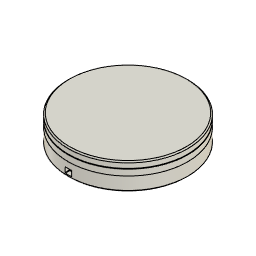
Turntable v8 (Autodesk Fusion 360 design; units mm, degrees)
Autodesk Fusion 360 part; units mm, degrees
sketch "Skizze1" plane through (0, 0, 0) normal (0, 0, 1) x (1, 0, 0)
  circle A0 centre (0, 0) radius 100
  circle A1 centre (0, 0) radius 86
  circle A2 centre (0, 0) radius 9
  dimension "d1" = 200
  dimension "d145" = 172
  dimension "d147" = 18
  constraint coincident A0.centre A1.centre
  constraint concentric A0 A2
  measures "d1" diameter of A0
  measures "d145" diameter of A1
  measures "d147" diameter of A2
extrude "Extrusion1" add sketch "Skizze1" along normal blind 10 from surface at 0.5 contours A0 | A1 | A2 makes body 1
chamfer "Fase1" distance 2 angle 45 1 edges at (-93.2327, -36.1615, 10.5) on bodies 1
sketch "Skizze2" plane through (0, 0, 0) normal (0, 1, 0) x (1, 0, 0)
  circle A0 centre (-93, 0) radius 3.5
  line L0 (0, 0) -> (-93, 0) construction
  dimension "d6" = 7
  dimension "d8" = 93
  constraint coincident L0.start origin
  constraint coincident A0.centre L0.end
  constraint horizontal L0
  measures "d6" diameter of A0
  measures "d8" distance of L0.start A0.centre
revolve "Drehen1" cut sketch "Skizze2" angle 360 about axis through (0, 0, 1.75) along (0, 0, 1) bodies 1
sketch "Skizze3" plane through (0, 0, 0) normal (0, 0, 1) x (1, 0, 0)
  circle A0 centre (0, 0) radius 100
  circle A1 centre (0, 0) radius 85
  line L0 (-3.8, 94) -> (-3.8, 91)
  arc A2 (-3.8, 91) -> (3.8, 91) centre (0, 91) ccw
  line L1 (3.8, 91) -> (3.8, 94)
  arc A3 (3.8, 94) -> (-3.8, 94) centre (0, 94) ccw
  line L2 (0, 94) -> (0, 91) construction
  line L3 (0, 0) -> (0, 94) construction
  line L4 (0, 0) -> (81.4064, 47) construction
  line L5 (79.5064, 50.2909) -> (76.9083, 48.7909)
  arc A4 (76.9083, 48.7909) -> (80.7083, 42.2091) centre (78.8083, 45.5) ccw
  line L6 (80.7083, 42.2091) -> (83.3064, 43.7091)
  arc A5 (83.3064, 43.7091) -> (79.5064, 50.2909) centre (81.4064, 47) ccw
  line L7 (81.4064, 47) -> (78.8083, 45.5) construction
  line L8 (0, 0) -> (81.4064, -47) construction
  line L9 (0, 0) -> (0, -94) construction
  line L10 (0, 0) -> (-81.4064, -47) construction
  line L11 (0, 0) -> (-81.4064, 47) construction
  line L12 (83.3064, -43.7091) -> (80.7083, -42.2091)
  arc A6 (80.7083, -42.2091) -> (76.9083, -48.7909) centre (78.8083, -45.5) ccw
  line L13 (76.9083, -48.7909) -> (79.5064, -50.2909)
  arc A7 (79.5064, -50.2909) -> (83.3064, -43.7091) centre (81.4064, -47) ccw
  line L14 (81.4064, -47) -> (78.8083, -45.5) construction
  line L15 (3.8, -94) -> (3.8, -91)
  arc A8 (3.8, -91) -> (-3.8, -91) centre (0, -91) ccw
  line L16 (-3.8, -91) -> (-3.8, -94)
  arc A9 (-3.8, -94) -> (3.8, -94) centre (0, -94) ccw
  line L17 (0, -94) -> (0, -91) construction
  line L18 (-79.5064, -50.2909) -> (-76.9083, -48.7909)
  arc A10 (-76.9083, -48.7909) -> (-80.7083, -42.2091) centre (-78.8083, -45.5) ccw
  line L19 (-80.7083, -42.2091) -> (-83.3064, -43.7091)
  arc A11 (-83.3064, -43.7091) -> (-79.5064, -50.2909) centre (-81.4064, -47) ccw
  line L20 (-81.4064, -47) -> (-78.8083, -45.5) construction
  line L21 (-83.3064, 43.7091) -> (-80.7083, 42.2091)
  arc A12 (-80.7083, 42.2091) -> (-76.9083, 48.7909) centre (-78.8083, 45.5) ccw
  line L22 (-76.9083, 48.7909) -> (-79.5064, 50.2909)
  arc A13 (-79.5064, 50.2909) -> (-83.3064, 43.7091) centre (-81.4064, 47) ccw
  line L23 (-81.4064, 47) -> (-78.8083, 45.5) construction
  dimension "d10" = 200
  dimension "d11" = 170
  dimension "d138" = 3.8
  dimension "d139" = 3
  dimension "d140" = 94
  dimension "d141" = 60
  dimension "d142" = 60
  constraint coincident A0.centre A1.centre
  constraint tangent L0 A2
  constraint tangent A2 L1
  constraint parallel L0 L1
  constraint tangent L1 A3
  constraint tangent L0 A3
  constraint coincident A3.centre L2.start
  constraint coincident A2.centre L3
  constraint vertical L3
  constraint tangent L5 A4
  constraint tangent A4 L6
  constraint parallel L5 L6
  constraint tangent L6 A5
  constraint tangent L5 A5
  constraint coincident L4 A4.centre
  constraint parallel L4 L7
  constraint coincident L4.end A5.centre
  constraint equal L1 L5
  constraint equal A3 A5
  constraint equal L3 L4
  constraint parallel L3 L9
  constraint parallel L8 L11
  constraint parallel L4 L10
  constraint equal L4 L8
  constraint equal L8 L9
  constraint equal L9 L10
  constraint equal L10 L11
  constraint tangent L12 A6
  constraint tangent A6 L13
  constraint parallel L12 L13
  constraint tangent L13 A7
  constraint tangent L12 A7
  constraint coincident L8 A6.centre
  constraint parallel L8 L14
  constraint coincident L8.end A7.centre
  constraint tangent L15 A8
  constraint tangent A8 L16
  constraint parallel L15 L16
  constraint tangent L16 A9
  constraint tangent L15 A9
  constraint coincident L9 A8.centre
  constraint parallel L9 L17
  constraint coincident L9.end A9.centre
  constraint tangent L18 A10
  constraint tangent A10 L19
  constraint parallel L18 L19
  constraint tangent L19 A11
  constraint tangent L18 A11
  constraint coincident L10 A10.centre
  constraint parallel L10 L20
  constraint coincident L10.end A11.centre
  constraint tangent L21 A12
  constraint tangent A12 L22
  constraint parallel L21 L22
  constraint tangent L22 A13
  constraint tangent L21 A13
  constraint coincident L11 A12.centre
  constraint parallel L11 L23
  constraint coincident L11.end A13.centre
  constraint equal A3 A13
  constraint equal A11 A13
  constraint equal A9 A11
  constraint equal A7 A9
  constraint equal L6 L12
  constraint equal L13 L15
  constraint equal L16 L18
  constraint equal L19 L21
  measures "d10" diameter of A0
  measures "d11" diameter of A1
  measures "d138" radius of A3
  measures "d139" distance of A2.end L1.end
  measures "d140" distance of A0.centre A3.centre
  measures "d141" angle of L3 L4
  measures "d142" angle of L4 L8
extrude "Extrusion3" add sketch "Skizze1" against normal blind 10 from surface at -0.5 separate body contours A0 | A1 | A2 makes body 2
revolve "Drehen2" cut sketch "Skizze2" angle 360 about axis through (0, 0, 1.75) along (0, 0, 1) bodies 2
sketch "Skizze4" plane through (0, 0, -0.5) normal (0, 0, 1) x (-1, 0, 0)
  circle A0 centre (0, 0) radius 89.5359
  circle A1 centre (0, 0) radius 4.9
  circle A2 centre (-17.5, -8) radius 2.1
  circle A3 centre (17.5, -8) radius 2.1
  line L0 (-17.5, -8) -> (17.5, -8) construction
  line L1 (0, 0) -> (0, -8) construction
  circle A4 centre (0, 0) radius 10
  circle A5 centre (17.5, -8) radius 3.7
  circle A6 centre (-17.5, -8) radius 3.7
  circle A7 centre (0, -86) radius 2.2
  line L2 (0, 0) -> (0, -86) construction
  line L3 (0, 0) -> (-74.4782, 43) construction
  line L4 (0, 0) -> (74.4782, 43) construction
  circle A8 centre (-74.4782, 43) radius 2.2
  circle A9 centre (74.4782, 43) radius 2.2
  circle A10 centre (0, 0) radius 83.8
  circle A11 centre (0, 0) radius 80
  dimension "d24" = 9.8
  dimension "d25" = 4.2
  dimension "d26" = 35
  dimension "d27" = 8
  dimension "d28" = 20
  dimension "d29" = 7.4
  dimension "d36" = 4.4
  dimension "d37" = 86
  dimension "d38" = 120
  dimension "d39" = 120
  dimension "d150" = 167.6
  dimension "d151" = 160
  constraint coincident A0.centre A1.centre
  constraint equal A2 A3
  constraint coincident A2.centre L0.start
  constraint coincident A3.centre L0.end
  constraint horizontal L0
  constraint midpoint L0 L1.end
  constraint vertical L1
  constraint concentric A3 A5
  constraint concentric A2 A6
  constraint equal A5 A6
  constraint coincident A7.centre L2.end
  constraint parallel L1 L2
  constraint equal L2 L3
  constraint equal L3 L4
  constraint coincident L3.end A8.centre
  constraint coincident L4.end A9.centre
  constraint equal A7 A8
  constraint equal A8 A9
  constraint concentric A4 A11
  measures "d24" diameter of A1
  measures "d25" diameter of A3
  measures "d26" distance of A2.centre A3.centre
  measures "d27" distance of A0.centre L1.end
  measures "d28" diameter of A4
  measures "d29" diameter of A5
  measures "d36" diameter of A7
  measures "d37" distance of A0.centre A7.centre
  measures "d38" angle of L2 L3
  measures "d39" angle of L3 L4
  measures "d150" diameter of A10
  measures "d151" diameter of A11
extrude "Extrusion4" cut sketch "Skizze4" against normal blind 10 contours A1 | A2 | A3 bodies 2
extrude "Extrusion5" cut sketch "Skizze4" against normal blind 8 contours A4 bodies 2
extrude "Extrusion6" cut sketch "Skizze4" against normal blind 4 contours A5 | A6 bodies 2
extrude "Extrusion7" cut sketch "Skizze4" against normal blind 10 contours A7 | A8 | A9 bodies 2
sketch "Skizze5" plane through (0, 0, 0.5) normal (0, 0, -1) x (1, 0, 0)
  circle A0 centre (0, 0) radius 89.5359
  circle A1 centre (0, 0) radius 9
  circle A2 centre (0, 0) radius 2.7
  line L0 (-1.6, 2.1749) -> (-1.6, -2.1749)
  line L1 (1.6, 2.1749) -> (1.6, -2.1749)
  dimension "d47" = 5.4
  dimension "d48" = 3.2
  dimension "d146" = 18
  constraint coincident A0.centre A1.centre
  constraint concentric A1 A2
  constraint coincident A2 L0.start
  constraint coincident A2 L0.end
  constraint vertical L0
  constraint coincident A2 L1.start
  constraint coincident A2 L1.end
  constraint parallel L0 L1
  constraint equal L0 L1
  measures "d47" diameter of A2
  measures "d48" distance of L0.start L1.start
  measures "d146" diameter of A1
extrude "Extrusion9" add sketch "Skizze5" along normal blind 8 contours A1 bodies 1
extrude "Extrusion10" add sketch "Skizze5" along normal blind 6.5 contours A2 L1 | A2 L0 bodies 1
sketch "Skizze6" plane through (0, 0, -10.5) normal (0, 0, -1) x (1, 0, 0)
  circle A0 centre (0, -86) radius 2.2
  circle A1 centre (74.4782, 43) radius 2.2
  circle A2 centre (-74.4782, 43) radius 2.2
  circle A3 centre (17.5, -8) radius 2.1
  circle A4 centre (0, 0) radius 4.9
  circle A5 centre (-17.5, -8) radius 2.1
  circle A6 centre (0, 0) radius 100
  circle A7 centre (0, 0) radius 97
  circle A8 centre (0, 0) radius 94
  dimension "d53" = 194
  dimension "d54" = 188
  constraint concentric A4 A7
  constraint coincident A4.centre A6.centre
  measures "d53" diameter of A7
  measures "d54" diameter of A8
extrude "Extrusion11" cut sketch "Skizze6" against normal blind 0.8 contours A7 bodies 2
chamfer "Fase2" distance 0.3 angle 45 2 edges at (-90.4358, -35.0767, -9.7) (-87.6388, 33.9919, -9.7) on bodies 2
ref_plane "Arbeitsebene1" through (0, 0, -10.5) normal (0, 0, 1) x (1, 0, 0)
sketch "Skizze7" plane through (0, 0, -10.5) normal (0, 0, 1) x (1, 0, 0)
  circle A0 centre (0, 0) radius 100
  circle A1 centre (0, 0) radius 96.75
  circle A2 centre (0, 0) radius 94.25
  circle A3 centre (0, 0) radius 93
  line L0 (0, 0) -> (0, 86) construction
  circle A4 centre (0, 86) radius 2
  circle A5 centre (0, 86) radius 3.5
  line L1 (-5, 86) -> (-5, 92.8655)
  line L2 (5, 86) -> (5, 92.8655)
  arc A6 (-5, 86) -> (5, 86) centre (0, 86) ccw
  line L3 (0, 0) -> (-74.4782, -43) construction
  line L4 (0, 0) -> (74.4782, -43) construction
  circle A7 centre (74.4782, -43) radius 2
  circle A8 centre (74.4782, -43) radius 3.5
  circle A9 centre (-74.4782, -43) radius 2
  circle A10 centre (-74.4782, -43) radius 3.5
  line L5 (-76.9782, -38.6699) -> (-82.9239, -42.1026)
  line L6 (-71.9782, -47.3301) -> (-77.9239, -50.7629)
  arc A11 (-71.9782, -47.3301) -> (-76.9782, -38.6699) centre (-74.4782, -43) ccw
  line L7 (76.9782, -38.6699) -> (82.9239, -42.1026)
  line L8 (71.9782, -47.3301) -> (77.9239, -50.7629)
  arc A12 (76.9782, -38.6699) -> (71.9782, -47.3301) centre (74.4782, -43) ccw
  dimension "d59" = 200
  dimension "d60" = 193.5
  dimension "d61" = 188.5
  dimension "d62" = 186
  dimension "d63" = 86
  dimension "d64" = 4
  dimension "d65" = 7
  dimension "d66" = 10
  dimension "d67" = 120
  dimension "d68" = 120
  constraint coincident A0.centre A1.centre
  constraint vertical L0
  constraint coincident L0.end A4.centre
  constraint concentric A4 A5
  constraint concentric A4 A6
  constraint coincident A3 L1.end
  constraint tangent L1 A6
  constraint coincident A3 L2.end
  constraint tangent L2 A6
  constraint equal L0 L3
  constraint equal L3 L4
  constraint coincident L4.end A7.centre
  constraint concentric A7 A8
  constraint concentric A7 A12
  constraint coincident L3.end A9.centre
  constraint concentric A9 A10
  constraint concentric A9 A11
  constraint equal A4 A9
  constraint equal A5 A10
  constraint equal A6 A11
  constraint equal A4 A7
  constraint equal A5 A8
  constraint equal A6 A12
  constraint coincident A3 L5.end
  constraint tangent L5 A11
  constraint coincident A3 L6.end
  constraint tangent L6 A11
  constraint parallel L0 L1
  constraint parallel L0 L2
  constraint parallel L3 L5
  constraint parallel L3 L6
  constraint coincident A3 L7.end
  constraint coincident A3 L8.end
  constraint parallel L4 L7
  constraint parallel L4 L8
  constraint tangent L8 A12
  constraint tangent L7 A12
  measures "d59" diameter of A0
  measures "d60" diameter of A1
  measures "d61" diameter of A2
  measures "d62" diameter of A3
  measures "d63" distance of A0.centre L0.end
  measures "d64" diameter of A4
  measures "d65" diameter of A5
  measures "d66" diameter of A6
  measures "d67" angle of L0 L3
  measures "d68" angle of L0 L4
extrude "Extrusion17" add sketch "Skizze7" against normal blind 23 separate body contours A0 | A1 | A2 | A3 L1 L2 A6 L5 L6 A11 L7 L8 A12 | A3 L1 L2 A6 | A3 L7 L8 A12 | A3 L5 L6 A11 | A4 | A5 | A7 | A8 | A9 | A10 makes body 3
extrude "Extrusion18" cut sketch "Skizze7" against normal blind 20 contours A3 L1 L2 A6 L5 L6 A11 L7 L8 A12 bodies 3
extrude "Extrusion19" cut sketch "Skizze7" against normal blind 23 contours A4 | A7 | A9 bodies 3
extrude "Extrusion20" cut sketch "Skizze7" against normal blind 7 from surface at -16 contours A5 | A8 | A10 bodies 3
fillet "Abrundung2" radius 5 6 edges at (-5, 92.8655, -20.5) (5, 92.8655, -20.5) (-77.9239, -50.7629, -20.5) (-82.9239, -42.1026, -20.5) (82.9239, -42.1026, -20.5) (77.9239, -50.7629, -20.5) on bodies 3
chamfer "Fase4" distance 1.5 angle 45 3 edges at (-77.7413, -44.2657, -26.5) (71.215, -44.2657, -26.5) (-3.2631, 84.7343, -26.5) on bodies 3
chamfer "Fase5" distance 2 angle 45 1 edges at (-93.2327, 36.1615, -33.5) on bodies 3
extrude "Extrusion21" add sketch "Skizze7" along normal blind 0.6 contours A1 bodies 3
chamfer "Fase6" distance 0.3 angle 45 2 edges at (-90.2027, -34.9863, -9.9) (-87.8719, 34.0823, -9.9) on bodies 3
sketch "Skizze8" plane through (0, 0, -30.5) normal (0, 0, 1) x (-1, 0, 0)
  arc A0 (-74.7346, 55.3511) -> (-73.2166, 48.0451) centre (-70.7166, 52.3752) ccw
  line L0 (-73.2166, 48.0451) -> (-71.9782, 47.3301)
  arc A1 (-76.9782, 38.6699) -> (-71.9782, 47.3301) centre (-74.4782, 43) ccw
  line L1 (-76.9782, 38.6699) -> (-78.2166, 39.3849)
  arc A2 (-78.2166, 39.3849) -> (-85.3027, 37.0465) centre (-80.7166, 35.0547) ccw
  arc A3 (-85.3027, 37.0465) -> (-10.5682, -92.3976) centre (0, 0) ccw
  arc A4 (-10.5682, -92.3976) -> (-5, -87.43) centre (-10, -87.43) ccw
  line L2 (-5, -87.43) -> (-5, -86)
  arc A5 (5, -86) -> (-5, -86) centre (0, -86) ccw
  line L3 (5, -86) -> (5, -87.43)
  arc A6 (5, -87.43) -> (10.5682, -92.3976) centre (10, -87.43) ccw
  arc A7 (10.5682, -92.3976) -> (85.3027, 37.0465) centre (0, 0) ccw
  arc A8 (85.3027, 37.0465) -> (78.2166, 39.3849) centre (80.7166, 35.0547) ccw
  line L4 (78.2166, 39.3849) -> (76.9782, 38.6699)
  arc A9 (71.9782, 47.3301) -> (76.9782, 38.6699) centre (74.4782, 43) ccw
  line L5 (71.9782, 47.3301) -> (73.2166, 48.0451)
  arc A10 (73.2166, 48.0451) -> (74.7346, 55.3511) centre (70.7166, 52.3752) ccw
  arc A11 (74.7346, 55.3511) -> (-74.7346, 55.3511) centre (0, 0) ccw
  line L6 (0, 0) -> (77.9423, -45) construction
  line L7 (0, 0) -> (0, 100) construction
  line L8 (86.9423, -29.4115) -> (68.9423, -60.5885)
  line L9 (77.3622, -36.0048) -> (69.8622, -48.9952)
  line L10 (77.3622, -36.0048) -> (75.6301, -35.0048)
  line L11 (75.6301, -35.0048) -> (68.1301, -47.9952)
  line L12 (68.1301, -47.9952) -> (69.8622, -48.9952)
  line L13 (86.9423, -29.4115) -> (82.6122, -26.9115)
  line L14 (82.6122, -26.9115) -> (92.4801, -9.8197)
  line L15 (68.9423, -60.5885) -> (64.6122, -58.0885)
  line L16 (64.6122, -58.0885) -> (54.7442, -75.1803)
  line L17 (82.6122, -26.9115) -> (77.3622, -36.0048)
  line L18 (64.6122, -58.0885) -> (69.8622, -48.9952)
  dimension "d99" = 90
  dimension "d100" = 120
  dimension "d101" = 36
  dimension "d102" = 15
  dimension "d103" = 2
  dimension "d104" = 5
  dimension "d105" = 5
  constraint coincident A3.centre A7.centre
  constraint vertical L7
  constraint perpendicular L6 L8
  constraint coincident L6.end L8
  constraint midpoint L6.end L8
  constraint perpendicular L6 L9
  constraint symmetric L6 L9.start L9.end
  constraint perpendicular L9 L10
  constraint perpendicular L6 L11
  constraint perpendicular L11 L12
  constraint perpendicular L8 L13
  constraint coincident A7 L14.end
  constraint perpendicular L13 L14
  constraint perpendicular L8 L15
  constraint coincident A7 L16.end
  constraint perpendicular L15 L16
  constraint equal L13 L15
  measures "d99" distance of A3.centre L6.end
  measures "d100" angle of L6 L7
  measures "d101" distance of L8.start L8.end
  measures "d102" distance of L10.end L11.end
  measures "d103" distance of L9.start L10.end
  measures "d104" distance of L8.start L9
  measures "d105" distance of L8.start L13.end
extrude "Extrusion22" add sketch "Skizze8" along normal blind 12 contours A7 L8 L13 L14 L15 L16 bodies 3
extrude "Extrusion23" add sketch "Skizze8" along normal blind 6 contours L9 L10 L11 L12 bodies 3
extrude "Extrusion24" add sketch "Skizze8" along normal blind 5 contours L8 L9 L13 L15 L17 L18 bodies 3
chamfer "Fase7" distance 1.5 angle 45 1 edges at (-71.8801, 41.5, -24.5) on bodies 3
fillet "Abrundung3" radius 1.5 2 edges at (-77.3622, 36.0048, -28) (-69.8622, 48.9952, -28) on bodies 3
fillet "Abrundung4" radius 0.5 2 edges at (-75.6301, 35.0048, -28.25) (-68.1301, 47.9952, -28.25) on bodies 3
sketch "Skizze9" plane through (-77.9423, 45, 0) normal (0.866025, -0.5, 0) x (0.5, 0.866025, 0)
  line L0 (-18, -25.5) -> (18, -25.5)
  line L1 (18, -25.5) -> (18, -18.5)
  line L2 (18, -18.5) -> (-18, -18.5)
  line L3 (-18, -18.5) -> (-18, -25.5)
  line L4 (-12.5, -20.2, -14.6955) -> (12.5, -20.2, -14.6955)
  line L5 (12.5, -20.2, -14.6955) -> (12.5, -24, -14.6955)
  line L6 (12.5, -24, -14.6955) -> (-12.5, -24, -14.6955)
  line L7 (-12.5, -24, -14.6955) -> (-12.5, -20.2, -14.6955)
  line L8 (0, -30.5, 0) -> (0, -24, -14.6955) construction
  point P0 (0, -30.5)
  dimension "d117" = 25
  dimension "d118" = 3.8
  dimension "d119" = 1.5
extrude "Extrusion25" cut sketch "Skizze9" along normal blind 15 contours L4 L5 L6 L7 in plane through (-90.669, 52.3478, 0) normal (0.866025, -0.5, 0) bodies 3
sketch "Skizze10" plane through (0, 0, -30.5) normal (0, 0, 1) x (-1, 0, 0)
  arc A0 (69.1122, -50.2942) -> (68.5631, -48.2452) centre (67.8131, -49.5442) ccw
  arc A1 (68.3801, -47.5622) -> (68.5631, -48.2452) centre (68.8131, -47.8122) ccw
  line L0 (68.3801, -47.5622) -> (75.3801, -35.4378)
  arc A2 (76.0631, -35.2548) -> (75.3801, -35.4378) centre (75.8131, -35.6878) ccw
  arc A3 (76.0631, -35.2548) -> (78.1122, -34.7058) centre (76.8131, -33.9558) ccw
  line L1 (78.1122, -34.7058) -> (92.4801, -9.8197)
  arc A4 (92.4801, -9.8197) -> (85.3027, 37.0465) centre (0, 0) ccw
  arc A5 (85.3027, 37.0465) -> (78.2166, 39.3849) centre (80.7166, 35.0547) ccw
  line L2 (78.2166, 39.3849) -> (76.9782, 38.6699)
  arc A6 (71.9782, 47.3301) -> (76.9782, 38.6699) centre (74.4782, 43) ccw
  line L3 (71.9782, 47.3301) -> (73.2166, 48.0451)
  arc A7 (73.2166, 48.0451) -> (74.7346, 55.3511) centre (70.7166, 52.3752) ccw
  arc A8 (74.7346, 55.3511) -> (-74.7346, 55.3511) centre (0, 0) ccw
  arc A9 (-74.7346, 55.3511) -> (-73.2166, 48.0451) centre (-70.7166, 52.3752) ccw
  line L4 (-73.2166, 48.0451) -> (-71.9782, 47.3301)
  arc A10 (-76.9782, 38.6699) -> (-71.9782, 47.3301) centre (-74.4782, 43) ccw
  line L5 (-76.9782, 38.6699) -> (-78.2166, 39.3849)
  arc A11 (-78.2166, 39.3849) -> (-85.3027, 37.0465) centre (-80.7166, 35.0547) ccw
  arc A12 (-85.3027, 37.0465) -> (-10.5682, -92.3976) centre (0, 0) ccw
  arc A13 (-10.5682, -92.3976) -> (-5, -87.43) centre (-10, -87.43) ccw
  line L6 (-5, -87.43) -> (-5, -86)
  arc A14 (5, -86) -> (-5, -86) centre (0, -86) ccw
  line L7 (5, -86) -> (5, -87.43)
  arc A15 (5, -87.43) -> (10.5682, -92.3976) centre (10, -87.43) ccw
  arc A16 (10.5682, -92.3976) -> (54.7442, -75.1803) centre (0, 0) ccw
  line L8 (54.7442, -75.1803) -> (69.1122, -50.2942)
  line L9 (-10, 92.4608) -> (10, 92.4608)
  line L10 (-7.5, 90.8608) -> (7.5, 90.8608) construction
  line L11 (7.5, 90.8608) -> (7.5, 50.3608) construction
  line L12 (7.5, 50.3608) -> (-7.5, 50.3608) construction
  line L13 (-7.5, 50.3608) -> (-7.5, 90.8608) construction
  line L14 (0, 92.4608) -> (0, 90.8608) construction
  circle A17 centre (-7.5, 50.3608) radius 2
  circle A18 centre (7.5, 50.3608) radius 2
  line L15 (-5.5, 90.8608) -> (-5.5, 92.4608)
  line L16 (-9.5, 90.8608) -> (-9.5, 92.4608)
  line L17 (5.5, 90.8608) -> (5.5, 92.4608)
  line L18 (9.5, 90.8553) -> (9.5044, 92.4608)
  arc A19 (-9.5, 90.8608) -> (-5.5, 90.8608) centre (-7.5, 90.8608) ccw
  arc A20 (5.5, 90.8608) -> (9.5, 90.8553) centre (7.5, 90.8608) ccw
  dimension "d122" = 20
  dimension "d123" = 15
  dimension "d124" = 40.5
  dimension "d125" = 1.6
  dimension "d126" = 4
  constraint coincident A8 L9.end
  constraint horizontal L9
  constraint horizontal L10
  constraint vertical L11
  constraint horizontal L12
  constraint vertical L13
  constraint midpoint L9 L14.start
  constraint midpoint L10 L14.end
  constraint vertical L14
  constraint coincident L10.start L13.end
  constraint coincident L10.end L11.start
  constraint coincident L12.end L13.start
  constraint coincident L11.end L12.start
  constraint equal A19 A20
  constraint equal A18 A20
  constraint equal A17 A18
  constraint coincident L10 L15.start
  constraint coincident L9 L15.end
  constraint tangent L15 A19
  constraint tangent L16 A19
  constraint coincident L10 L17.start
  constraint coincident L9 L17.end
  constraint tangent L17 A20
  constraint coincident L9 L18.end
  constraint tangent L18 A20
  constraint coincident L9 L16.end
  constraint coincident A8 L9.start
  constraint perpendicular L9 L16
  measures "d122" distance of L9.start L9.end
  measures "d123" distance of L11.end L12.end
  measures "d124" distance of L10.end L11.end
  measures "d125" distance of L14.start L14.end
  measures "d126" diameter of A19
extrude "Extrusion26" add sketch "Skizze10" along normal blind 12 contours A8 L9 bodies 3
extrude "Extrusion27" add sketch "Skizze10" along normal blind 2.2 contours L9 L17 L18 A20 | L9 L15 L16 A19 | A17 | A18 bodies 3
sketch "Skizze11" plane through (0, -92.4608, 0) normal (0, 1, 0) x (-1, 0, 0)
  line L0 (-5.5, -28.3) -> (-5.5, -30.5)
  line L1 (-5.5, -30.5) -> (5.5, -30.5)
  line L2 (5.5, -30.5) -> (5.5, -28.3)
  line L3 (5.5, -28.3) -> (9.5044, -28.3)
  line L4 (9.5044, -28.3) -> (9.5044, -30.5)
  line L5 (9.5044, -30.5) -> (10, -30.5)
  line L6 (10, -30.5) -> (10, -18.5)
  line L7 (10, -18.5) -> (-10, -18.5)
  line L8 (-10, -18.5) -> (-10, -30.5)
  line L9 (-10, -30.5) -> (-9.5, -30.5)
  line L10 (-9.5, -30.5) -> (-9.5, -28.3)
  line L11 (-9.5, -28.3) -> (-5.5, -28.3)
  line L12 (-5.5, -20.5) -> (5.5, -20.5)
  line L13 (5.5, -20.5) -> (5.5, -29.5)
  line L14 (5.5, -29.5) -> (-5.5, -29.5)
  line L15 (-5.5, -29.5) -> (-5.5, -20.5)
  line L16 (0, 0) -> (0, -20.5) construction
  dimension "d131" = 11
  dimension "d132" = 9
  dimension "d133" = 20.5
  constraint horizontal L12
  constraint vertical L13
  constraint horizontal L14
  constraint vertical L15
  constraint coincident L16.start origin
  constraint midpoint L12 L16.end
  constraint vertical L16
  measures "d131" distance of L12.start L12.end
  measures "d132" distance of L12.start L14.end
  measures "d133" distance of L16.start L16.end
extrude "Extrusion28" cut sketch "Skizze11" against normal blind 8 contours L0 L2 L12 L13 L14 L15 bodies 3
chamfer "Fase8" distance 0.5 angle 45 2 edges at (-5.5, -96.1547, -20.5) (5.5, -96.1547, -20.5) on bodies 3
chamfer "Fase9" distance 0.5 angle 45 8 edges at (-5.5, -96.1547, -29.5) (-5.5, -91.6608, -30.5) (-9.5022, -91.658, -30.5) (-7.4972, -88.8608, -30.5) (5.5, -96.1547, -29.5) (5.5, -91.6608, -30.5) (7.5, -88.8608, -30.5) (9.5, -91.6608, -30.5) on bodies 3
extrude "Extrusion29" add sketch "Skizze3" along normal mid plane 0.6 separate body makes body 4
extrude "Extrusion30" cut sketch "Skizze1" along normal blind 4 contours A1 bodies 1
extrude "Extrusion31" add sketch "Skizze4" along normal blind 2 contours A10 bodies 2
chamfer "Fase10" distance 1 angle 45 2 edges at (78.129, 30.3034, 1.5) (74.5862, -28.9292, 1.5) on bodies 2
